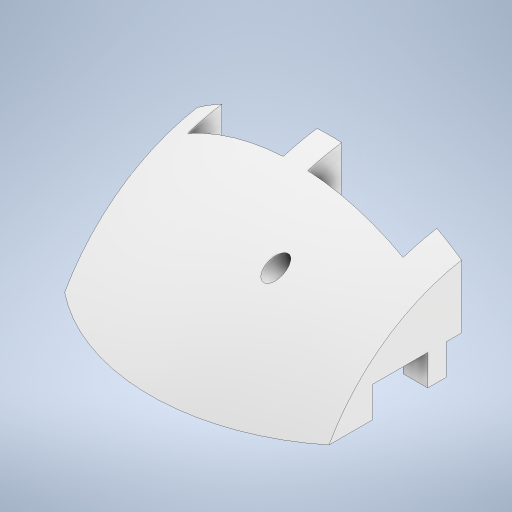
# Autodesk Inventor part: back back gabagaba
Saved by Autodesk Inventor 2023 (Build 270158000, 158)
## iProperties
Created: 2022-10-08
Part Number: back back gabagaba
Material: ABS プラスチック
Document SubType Name: Modeling
Designer: ellie
Density: 1.06 g/cm^3
Appearance: 積雪
Author: ellie
Autodesk Inventor part; units mm, degrees
sketch "スケッチ1" plane through (0, 0, 0) normal (0, 1, 0) x (-1, 0, 0)
  circle A0 centre (0, 0) radius 37.5
  line L0 (0, 0) -> (0, -37.5)
  line L1 (0, 0) -> (0, 37.5)
  dimension "d0" = 75
  constraints: 4 end point, 2 point on circle, 2 vertical, 1 centre point, 1 coincident
  measures "d0" diameter of A0
revolve "回転1" add sketch "スケッチ1" angle 180 about axis through (0, 0, 0) along (0, 0, 1) picked at (-2.7815, -24.6866) contours L1 L0 A0
sketch "スケッチ5" plane through (0, 0, 0) normal (0, -1, 0) x (1, 0, 0)
  line L0 (-21, -21) -> (21, -21)
  line L1 (21, -21) -> (21, -9)
  line L2 (21, -9) -> (-21, -9)
  line L3 (-21, -9) -> (-21, -21)
  line L4 (-21, -11) -> (-21, -9)
  line L5 (0, 25.75) -> (-17, 25.75)
  line L6 (-17, 25.75) -> (-17, 24.25)
  line L7 (-17, 24.25) -> (0, 24.25)
  line L8 (0, 24.25) -> (0, 25.75)
  line L9 (0, 22.75) -> (-20.5, 22.75)
  line L10 (-20.5, 22.75) -> (-20.5, 21.25)
  line L11 (-20.5, 21.25) -> (0, 21.25)
  line L12 (0, 21.25) -> (0, 22.75)
  line L13 (0, 15.75) -> (-21.5, 15.75)
  line L14 (-21.5, 15.75) -> (-21.5, 13.25)
  line L15 (-21.5, 13.25) -> (0, 13.25)
  line L16 (0, 13.25) -> (0, 15.75)
  line L17 (0, 7.75) -> (-22, 7.75)
  line L18 (-22, 7.75) -> (-22, 5.25)
  line L19 (-22, 5.25) -> (0, 5.25)
  line L20 (0, 5.25) -> (0, 7.75)
  circle A0 centre (0, 0) radius 37.5 projected
  circle A1 centre (0, 0) radius 37.5 projected
  line L21 (0, 37.5) -> (0, -37.5)
  line L22 (37.5, 0) -> (-37.5, 0)
  line L23 (-33.5, 5.25) -> (-24, 5.25)
  line L24 (-24, 5.25) -> (-24, -5.25)
  line L25 (-24, -5.25) -> (-33.5, -5.25)
  line L26 (-33.5, -5.25) -> (-33.5, 5.25)
  line L27 (-24, -8.0262) -> (-24, 5.25)
  line L28 (-29, 23.775) -> (-29, -23.775)
  line L29 (-14, 25.75) -> (0, 25.75)
  line L30 (0, 25.75) -> (0, 37.5)
  line L31 (-14, 37.5) -> (-14, 25.75)
  line L32 (-14, 24.25) -> (0, 24.25)
  line L33 (0, 24.25) -> (0, 22.75)
  line L34 (0, 22.75) -> (-14, 22.75)
  line L35 (-14, 22.75) -> (-14, 24.25)
  line L36 (-19, 15.75) -> (0, 15.75)
  line L37 (0, 15.75) -> (0, 21.25)
  line L38 (0, 21.25) -> (-19, 21.25)
  line L39 (-19, 21.25) -> (-19, 15.75)
  line L40 (-19, 13.25) -> (0, 13.25)
  line L41 (0, 13.25) -> (0, 7.75)
  line L42 (0, 7.75) -> (-19, 7.75)
  line L43 (-19, 7.75) -> (-19, 13.25)
  line L44 (-24, 0) -> (-40.9365, 0)
  line L45 (-24, 0) -> (-9.0837, 0)
  line L46 (-8.5, 5.25) -> (-24, 5.25)
  line L47 (-24, 5.25) -> (-24, -5.25)
  line L48 (-24, -5.25) -> (-8.5, -5.25)
  line L49 (-8.5, 5.25) -> (-24, -5.25) construction
  line L50 (-24, 5.25) -> (-8.5, -5.25) construction
  line L51 (-24, 7.25) -> (-34.5, 7.25)
  line L52 (-34.5, 7.25) -> (-34.5, -7.25)
  line L53 (-34.5, -7.25) -> (-24, -7.25)
  line L54 (-24, 7.25) -> (-34.5, -7.25) construction
  line L55 (-34.5, 7.25) -> (-24, -7.25) construction
  line L56 (-8.5, 5.25) -> (-1, 5.25)
  line L57 (-1, 5.25) -> (-1, -5.25)
  line L58 (-1, -5.25) -> (-8.5, -5.25)
  line L59 (-8.5, 5.25) -> (-1, -5.25) construction
  line L60 (-1, 5.25) -> (-8.5, -5.25) construction
  line L61 (-24, 5.25) -> (-29, 5.25)
  line L62 (-24, -5.25) -> (-29, -5.25)
  line L63 (-24, 7.25) -> (-29, 7.25)
  line L64 (-24, -7.25) -> (-29, -7.25)
  line L65 (27.0231, -26) -> (-27.0231, -26)
  line L66 (-8.5, 5.25) -> (-7.3, 5.25)
  line L67 (-7.3, -5.25) -> (-8.5, -5.25)
  line L68 (-4, 7.75) -> (-1, 7.75)
  line L69 (0, 22.75) -> (-4, 22.75)
  line L70 (-4, 21.25) -> (0, 21.25)
  line L71 (0, 21.25) -> (0, 22.75)
  line L72 (-7, 7.75) -> (-2, 7.75)
  line L73 (-1, 5.25) -> (-6.5, 5.25)
  line L74 (-24, 5.25) -> (-24, 7.25)
  point P0 (0, -21)
  point P1 (0, -9)
  point P2 (0, 25)
  point P3 (0, 22)
  point P4 (0, 14.5)
  point P5 (0, 6.5)
  point P6 (-21, -15)
  point P7 (-27, -0.5262)
  point P8 (-14, 23.5)
  point P9 (-14, 34.7886)
  point P10 (0, 25.75)
  point P11 (0, 24.25)
  point P12 (0, 13.25)
  point P13 (0, 15.75)
  point P14 (-29, 0)
  point P15 (-33.5, 0)
  point P16 (-24, 0)
  point P17 (-16.25, 0)
  point P18 (-29.25, 0)
  point P19 (-4.75, 0)
  point P20 (-27, 0.5)
  point P21 (-28, 0.4738)
  point P22 (-28, -11.5262)
  point P23 (-27, -11.5)
  point P24 (-24, 5.25)
  point P25 (-24, 5.25)
  point P26 (-1, 0)
  point P27 (0, 21.25)
  point P28 (0, 22.75)
  point P29 (-29, -7.25)
  point P30 (-29, 7.25)
  point P31 (-7.9, -5.25)
  point P32 (-7.9, 5.25)
  dimension "d12" = 42
  dimension "d13" = 12
  dimension "d23" = 17
  dimension "d24" = 1.5
  dimension "d27" = 20.5
  dimension "d28" = 1.5
  dimension "d30" = 21.5
  dimension "d31" = 2.5
  dimension "d33" = 2.5
  dimension "d88" = 0
  dimension "d89" = 0
  dimension "d90" = 16.5
  dimension "d92" = 21
  dimension "d97" = 9.5
  dimension "d98" = 10.5
  dimension "d113" = 29
  dimension "d122" = 14
  dimension "d124" = 1.5
  dimension "d125" = 14
  dimension "d126" = 5.5
  dimension "d127" = 5.5
  dimension "d128" = 19
  dimension "d129" = 19
  dimension "d161" = 14.5
  dimension "d162" = 10.5
  dimension "d164" = 10.5
  dimension "d170" = 26
  dimension "d326" = 23
  dimension "d327" = 10.5
  dimension "d329" = 15.5
  dimension "d330" = 34.5
  dimension "d359" = 22
  constraints: 148 end point, 26 parallel, 20 horizontal, 17 midpoint, 17 perpendicular, 16 point on line, 9 collinear, 2 vertical, 20 other
  measures "d12" distance of L2.end L1.end
  measures "d13" distance of L1.end L0.end
  measures "d23" distance of L7.end L6.end
  measures "d24" distance of L6.end L5.end
  measures "d27" distance of L11.end L10.end
  measures "d28" distance of L10.end L9.end
  measures "d30" distance of L15.end L14.end
  measures "d31" distance of L14.end L13.end
  measures "d33" distance of L18.end L17.end
  measures "d89" distance from line of point (0, 0) L22
  measures "d90" distance from line of L0 point (0, -37.5)
  measures "d92" distance of the line from the sketch origin of L3
  measures "d97" distance of L24.end L25.end
  measures "d98" distance of L23.end L24.end
  measures "d113" distance of the line from the sketch origin of L28
  measures "d122" distance of the line from the sketch origin of L31
  measures "d124" distance of L32.end L33.end
  measures "d126" distance of L37.end L36.end
  measures "d127" distance of L40.end L41.end
  measures "d128" distance of the line from the sketch origin of L43
  measures "d129" distance of the line from the sketch origin of L39
  measures "d161" distance between parallel lines of L53 L51
  measures "d162" distance between parallel lines of L47 L52
  measures "d164" distance between parallel lines of L58 L56
  measures "d170" distance between parallel lines of L65 L22
  measures "d326" distance between parallel lines of L47 L57
  measures "d327" distance between parallel lines of L48 L46
  measures "d329" distance of L47.end L48.end
  measures "d330" distance of the line from the sketch origin of L52
  measures "d359" distance of the line from the sketch origin of L18
extrude "GNSボード" cut sketch "スケッチ5" against normal blind 16 contours L8 L7 L6 L5
extrude "GNSボード止めるよう" cut sketch "スケッチ5" against normal blind 15 contours L21 L5 L31 A0 | L21 L9 L35 L7
extrude "アルミ板１" cut sketch "スケッチ5" against normal blind 20 contours L11 L10 L9 L12
extrude "メイン基板" cut sketch "スケッチ5" against normal blind 20 contours L15 L14 L13 L16
extrude "メイン止めるよう" cut sketch "スケッチ5" against normal blind 15 contours L17 L43 L15 L21 | L13 L39 L11 L21
extrude "アルミ板２" cut sketch "スケッチ5" against normal blind 20 contours L19 L18 L17 L20
extrude "電池ボックス入れ" cut sketch "スケッチ5" against normal blind 13 contours L3 L2 L21 L0 | L21 L2 L1 L0
extrude "side ut" cut sketch "スケッチ5" against normal blind 100 contours A0 L22 L52 L53 L28 | A0 L28 L51 L52 L22 | L53 L52 L22 L26 L25 L28 | L52 L51 L28 L23 L26 L22 | L25 L26 L22 L28 | L22 L26 L23 L28
extrude "motor case" add sketch "スケッチ5" against normal blind 7 contours L53 L52 L22 L26 L25 L28 | L24 L25 L28 L22 | L22 L28 L23 L24 | L52 L51 L28 L23 L26 L22 | L25 L26 L22 L28 | L22 L26 L23 L28
extrude "bottom cut" cut sketch "スケッチ5" against normal blind 90 contours L65 A0 L21 | L21 A0 L65
extrude "motor" cut sketch "スケッチ5" against normal blind 6 contours L57 L58 L48 L24 L22 | L22 L24 L46 L19 L57 | L24 L25 L28 L22 | L22 L28 L23 L24 | L25 L26 L22 L28 | L22 L26 L23 L28
sketch "スケッチ27" plane through (-34.5, 0, -7.25) normal (-1, 0, 0) x (0, 0, 1)
  line L0 (14.5, 0) -> (0, 0) projected
  circle A0 centre (7.25, 0) radius 3
  point P0 (7.25, 0)
  dimension "d198" = 6
  constraints: 1 centre point, 1 midpoint
  measures "d198" diameter of A0
extrude "moter shaft" cut sketch "スケッチ27" against normal blind 27
mirror "ミラー13" about plane through (0, 0, 0) normal (1, 0, 0) of "メイン止めるよう", "メイン基板", "アルミ板１", "GNSボード止めるよう", "GNSボード", "アルミ板２", "motor", "motor case", "moter shaft", "電池ボックス入れ", "side ut"
ref_plane "作業平面5" through (-17, 17.5, 24.25) normal (0, -1, 0) x (1, 0, 0)
ref_plane "作業平面6" through (21, 13, -9) normal (0, 0, -1) x (1, 0, 0)
ref_plane "作業平面7" through (29, 35, 7.25) normal (0, -1, 0) x (1, 0, 0)
sketch "スケッチ41" plane through (-17, 0, 24.25) normal (0, -1, 0) x (1, 0, 0)
  line L0 (-17.5, -21.25) -> (-16.5, -21.25) projected
  line L1 (-16.5, -21.25) -> (-16.5, -19) projected
  line L2 (-16.5, -19) -> (-5, -19) projected
  line L3 (-5, -19) -> (-5, -16.5) projected
  line L4 (-5, -16.5) -> (-2, -16.5) projected
  line L5 (-2, -16.5) -> (-2, -11) projected
  line L6 (-2, -11) -> (-4.5, -11) projected
  line L7 (-4.5, -11) -> (-4.5, -8.5) projected
  line L8 (-4.5, -8.5) -> (-2, -8.5) projected
  line L9 (-2, -8.5) -> (-2, -3) projected
  line L10 (-2, -3) -> (-3.5, -3) projected
  line L11 (-3.5, -3) -> (-3.5, -1.5) projected
  line L12 (-3.5, -1.5) -> (3, -1.5) projected
  line L13 (3, -1.5) -> (3, 0) projected
  line L14 (3, 0) -> (0, 0) projected
  line L15 (0, 0) -> (0, 1.5) projected
  line L16 (0, 1.5) -> (3, 1.5) projected
  line L17 (3, 1.5) -> (3, 10.5386) projected
  arc A0 (3, 10.5386) -> (-12, -0.475) centre (17, -24.25) ccw projected
  line L18 (-12, -0.475) -> (-12, -17) projected
  line L19 (-12, -17) -> (-17.5, -17) projected
  line L20 (-17.5, -17) -> (-17.5, -21.25) projected
  line L21 (-2, -16.5) -> (-2, -11) projected
  line L22 (-4.5, -8.5) -> (-4.5, -11) projected
  line L23 (0, 1.5) -> (0, 0) projected
  circle A1 centre (-4.5, 2.5) radius 2.25
  dimension "d252" = 4.5
  dimension "d253" = 4.5
  dimension "d254" = 4
  constraints: 1 centre point
  measures "d252" diameter of A1
  measures "d253" distance from line of A1.centre L15
  measures "d254" distance from line of A1.centre L12
extrude "top lock 10mm" cut sketch "スケッチ41" against normal blind 3 contours A1
mirror "ミラー15" about plane through (0, 0, 0) normal (1, 0, 0) of "top lock 10mm"
sketch "スケッチ42" plane through (-34.5, 0, -7.25) normal (0, -1, 0) x (1, 0, 0)
  circle A0 centre (9.5, -14) radius 2.25
  line L0 (13.5, -13.75) -> (13.5, -1.75) projected
  line L1 (33.5, 2) -> (1, 2) projected
  point P0 (34.5, 7.25)
  point P1 (10, 2)
  point P2 (7.8183, 2)
  point P3 (12.1817, 2)
  dimension "d257" = 4
  dimension "d258" = 4.5
  dimension "d259" = 16
  constraints: 1 centre point
  measures "d257" distance from line of A0.centre L0
  measures "d258" diameter of A0
  measures "d259" distance from line of A0.centre L1
extrude "bottom lock" cut sketch "スケッチ42" against normal blind 3
mirror "ミラー16" about plane through (0, 0, 0) normal (1, 0, 0) of "bottom lock"
ref_plane "作業平面8" through (-17, 15, 24.25) normal (0, -1, 0) x (1, 0, 0)
sketch "スケッチ45" plane through (-17, 15, 24.25) normal (0, -1, 0) x (1, 0, 0)
  circle A0 centre (-4.5, 2.5) radius 2.25 projected
  line L0 (-17.5, -21.25) -> (-16.5, -21.25) projected
  line L1 (-16.5, -21.25) -> (-16.5, -19) projected
  line L2 (-16.5, -19) -> (-5, -19) projected
  line L3 (-5, -19) -> (-5, -16.5) projected
  line L4 (-5, -16.5) -> (-2, -16.5) projected
  line L5 (-2, -16.5) -> (-2, -11) projected
  line L6 (-2, -11) -> (-4.5, -11) projected
  line L7 (-4.5, -11) -> (-4.5, -8.5) projected
  line L8 (-4.5, -8.5) -> (-2, -8.5) projected
  line L9 (-2, -8.5) -> (-2, -3) projected
  line L10 (-2, -3) -> (-3.5, -3) projected
  line L11 (-3.5, -3) -> (-3.5, -1.5) projected
  line L12 (-3.5, -1.5) -> (3, -1.5) projected
  line L13 (3, -1.5) -> (3, 0) projected
  line L14 (3, 0) -> (0, 0) projected
  line L15 (0, 0) -> (0, 1.5) projected
  line L16 (0, 1.5) -> (3, 1.5) projected
  line L17 (3, 1.5) -> (3, 10.5386) projected
  arc A1 (3, 10.5386) -> (-12, -0.475) centre (17, -24.25) ccw projected
  line L18 (-12, -0.475) -> (-12, -17) projected
  line L19 (-12, -17) -> (-17.5, -17) projected
  line L20 (-17.5, -17) -> (-17.5, -21.25) projected
  arc A2 (31, 7.1387) -> (3, 7.1387) centre (17, -24.25) ccw projected
  line L21 (3, 1.5) -> (3, 7.1387) projected
  line L22 (31, 1.5) -> (3, 1.5) projected
  line L23 (31, 1.5) -> (31, 7.1387) projected
  circle A3 centre (38.5, 2.5) radius 2.25 projected
  line L24 (50.5, -21.25) -> (51.5, -21.25) projected
  line L25 (51.5, -17) -> (51.5, -21.25) projected
  line L26 (46, -17) -> (51.5, -17) projected
  line L27 (46, -17) -> (46, -0.475) projected
  arc A4 (46, -0.475) -> (31, 10.5386) centre (17, -24.25) ccw projected
  line L28 (31, 10.5386) -> (31, 1.5) projected
  line L29 (31, 1.5) -> (34, 1.5) projected
  line L30 (34, 1.5) -> (34, 0) projected
  line L31 (34, 0) -> (31, 0) projected
  line L32 (31, 0) -> (31, -1.5) projected
  line L33 (31, -1.5) -> (37.5, -1.5) projected
  line L34 (37.5, -1.5) -> (37.5, -3) projected
  line L35 (37.5, -3) -> (36, -3) projected
  line L36 (36, -3) -> (36, -8.5) projected
  line L37 (36, -8.5) -> (38.5, -8.5) projected
  line L38 (38.5, -8.5) -> (38.5, -11) projected
  line L39 (38.5, -11) -> (36, -11) projected
  line L40 (36, -11) -> (36, -16.5) projected
  line L41 (36, -16.5) -> (39, -16.5) projected
  line L42 (39, -16.5) -> (39, -19) projected
  line L43 (39, -19) -> (50.5, -19) projected
  line L44 (50.5, -19) -> (50.5, -21.25) projected
  circle A5 centre (38.5, 2.5) radius 2.25 projected
  arc A6 (-17.5, -21.25) -> (-17.5, -21.25) centre (-4.5, 2.5) ccw projected
  line L45 (34, 0) -> (0, 0) projected
  line L46 (34, 0) -> (34, 1.5) projected
  line L47 (34, 1.5) -> (0, 1.5) projected
  line L48 (0, 0) -> (0, 1.5) projected
  line L49 (31, -1.5) -> (3, -1.5) projected
  line L50 (31, -1.5) -> (31, 0) projected
  line L51 (3, 0) -> (31, 0) projected
  line L52 (3, -1.5) -> (3, 0) projected
  line L53 (-2, -3) -> (36, -3) projected
  arc A7 (50.5, -21.25) -> (50.5, -21.25) centre (38.5, 2.5) ccw projected
  line L54 (36, -8.5) -> (-2, -8.5) projected
  line L55 (36, -8.5) -> (36, -3) projected
  line L56 (-2, -3) -> (36, -3) projected
  line L57 (-2, -8.5) -> (-2, -3) projected
  line L58 (-2, -11) -> (36, -11) projected
  line L59 (36, -16.5) -> (-2, -16.5) projected
  line L60 (36, -16.5) -> (36, -11) projected
  line L61 (-2, -11) -> (36, -11) projected
  line L62 (-2, -16.5) -> (-2, -11) projected
  line L63 (39, -19) -> (-5, -19) projected
  line L64 (39, -19) -> (39, -16.5) projected
  line L65 (39, -16.5) -> (-5, -16.5) projected
  line L66 (-5, -19) -> (-5, -16.5) projected
  line L67 (-5, -19) -> (16, -19) projected
  line L68 (-16.5, -19) -> (-5, -19) projected
  line L69 (-16.5, -29.5) -> (-16.5, -19) projected
  line L70 (16, -29.5) -> (-16.5, -29.5) projected
  circle A8 centre (42, -45.5) radius 2.25 projected
  circle A9 centre (-8, -45.5) radius 2.25 projected
  line L71 (18, -29.5) -> (18, -19) projected
  line L72 (18, -19) -> (16, -19) projected
  line L73 (16, -19) -> (16, -29.5) projected
  line L74 (-5, -19) -> (-5, -16.5) projected
  line L75 (-16.5, -29.5) -> (-16.5, -27.25) projected
  line L76 (-16.5, -27.25) -> (-17.5, -27.25) projected
  line L77 (-17.5, -27.25) -> (-17.5, -31.5) projected
  line L78 (-17.5, -31.5) -> (-12, -31.5) projected
  line L79 (-12, -31.5) -> (-12, -48.025) projected
  arc A10 (-12, -48.025) -> (-10.0231, -50.25) centre (17, -24.25) ccw projected
  line L80 (-10.0231, -50.25) -> (44.0231, -50.25) projected
  arc A11 (44.0231, -50.25) -> (46, -48.025) centre (17, -24.25) ccw projected
  line L81 (46, -48.025) -> (46, -31.5) projected
  line L82 (51.5, -31.5) -> (46, -31.5) projected
  line L83 (51.5, -27.25) -> (51.5, -31.5) projected
  line L84 (51.5, -27.25) -> (50.5, -27.25) projected
  line L85 (50.5, -27.25) -> (50.5, -29.5) projected
  line L86 (39, -16.5) -> (39, -19) projected
  line L87 (-4, -33.25) -> (38, -33.25) projected
  line L88 (38, -33.25) -> (38, -45.25) projected
  line L89 (38, -45.25) -> (-4, -45.25) projected
  line L90 (-4, -45.25) -> (-4, -33.25) projected
  line L91 (-5, -13.5) -> (39, -13.5)
  line L92 (39, -13.5) -> (39, 10.1193)
  line L93 (39, 10.1193) -> (-5, 10.1193)
  line L94 (-5, 10.1193) -> (-5, -13.5)
  line L95 (16, -19) -> (16, -29.5) projected
  line L96 (-17.5, -21.25) -> (-16.5, -21.25) projected
  line L97 (-16.5, -21.25) -> (-16.5, -19) projected
  line L98 (-16.5, -19) -> (-5, -19) projected
  line L99 (-5, -16.5) -> (-2, -16.5) projected
  line L100 (-2, -16.5) -> (-2, -11) projected
  line L101 (-2, -11) -> (-4.5, -11) projected
  line L102 (-4.5, -11) -> (-4.5, -8.5) projected
  line L103 (-4.5, -8.5) -> (-2, -8.5) projected
  line L104 (-2, -8.5) -> (-2, -3) projected
  line L105 (-2, -3) -> (-3.5, -3) projected
  line L106 (-3.5, -3) -> (-3.5, -1.5) projected
  line L107 (-3.5, -1.5) -> (3, -1.5) projected
  line L108 (3, -1.5) -> (3, 0) projected
  line L109 (3, 0) -> (0, 0) projected
  line L110 (0, 0) -> (0, 1.5) projected
  line L111 (0, 1.5) -> (3, 1.5) projected
  line L112 (3, 1.5) -> (3, 10.5386) projected
  line L113 (-12, -0.475) -> (-12, -17) projected
  line L114 (-12, -17) -> (-17.5, -17) projected
  line L115 (-17.5, -17) -> (-17.5, -21.25) projected
  line L116 (16, -29.5) -> (-16.5, -29.5) projected
  line L117 (50.5, -29.5) -> (18, -29.5) projected
  line L118 (50.5, -21.25) -> (51.5, -21.25) projected
  line L119 (51.5, -17) -> (51.5, -21.25) projected
  line L120 (46, -17) -> (51.5, -17) projected
  line L121 (46, -17) -> (46, -0.475) projected
  line L122 (31, 10.5386) -> (31, 1.5) projected
  line L123 (31, 1.5) -> (34, 1.5) projected
  line L124 (34, 1.5) -> (34, 0) projected
  line L125 (34, 0) -> (31, 0) projected
  line L126 (31, 0) -> (31, -1.5) projected
  line L127 (31, -1.5) -> (37.5, -1.5) projected
  line L128 (37.5, -1.5) -> (37.5, -3) projected
  line L129 (37.5, -3) -> (36, -3) projected
  line L130 (36, -3) -> (36, -8.5) projected
  line L131 (36, -8.5) -> (38.5, -8.5) projected
  line L132 (38.5, -8.5) -> (38.5, -11) projected
  line L133 (38.5, -11) -> (36, -11) projected
  line L134 (36, -11) -> (36, -16.5) projected
  line L135 (36, -16.5) -> (39, -16.5) projected
  line L136 (39, -19) -> (50.5, -19) projected
  line L137 (50.5, -19) -> (50.5, -21.25) projected
  arc A12 (3, 10.5386) -> (-12, -0.475) centre (17, -24.25) ccw projected
  arc A13 (46, -0.475) -> (31, 10.5386) centre (17, -24.25) ccw projected
  arc A14 (44.0231, -50.25) -> (46, -48.025) centre (17, -24.25) ccw projected
  arc A15 (-12, -48.025) -> (-10.0231, -50.25) centre (17, -24.25) ccw projected
  circle A16 centre (-4.5, 2.5) radius 2.25 projected
  circle A17 centre (38.5, 2.5) radius 2.25 projected
  line L138 (51.5, -27.25) -> (50.5, -27.25) projected
  line L139 (50.5, -29.5) -> (18, -29.5) projected
  line L140 (18, -29.5) -> (18, -19) projected
  line L141 (18, -19) -> (16, -19) projected
  line L142 (16, -19) -> (16, -29.5) projected
  line L143 (16, -29.5) -> (-16.5, -29.5) projected
  line L144 (-17.5, -21.25) -> (-16.5, -21.25) projected
  line L145 (-16.5, -27.25) -> (-17.5, -27.25) projected
  line L146 (-16.5, -29.5) -> (-16.5, -27.25) projected
  line L147 (-17.5, -27.25) -> (-17.5, -31.5) projected
  line L148 (-17.5, -31.5) -> (-12, -31.5) projected
  line L149 (-12, -31.5) -> (-12, -48.025) projected
  arc A18 (-12, -48.025) -> (-10.0231, -50.25) centre (17, -24.25) ccw projected
  line L150 (-10.0231, -50.25) -> (44.0231, -50.25) projected
  line L151 (46, -48.025) -> (46, -31.5) projected
  line L152 (51.5, -31.5) -> (46, -31.5) projected
  line L153 (51.5, -27.25) -> (51.5, -31.5) projected
  line L154 (50.5, -27.25) -> (50.5, -29.5) projected
  line L155 (51.5, -27.25) -> (50.5, -27.25) projected
  line L156 (50.5, -21.25) -> (51.5, -21.25) projected
  line L157 (50.5, -29.5) -> (18, -29.5) projected
  line L158 (18, -29.5) -> (18, -19) projected
  line L159 (18, -19) -> (16, -19) projected
  line L160 (16, -19) -> (16, -29.5) projected
  line L161 (16, -29.5) -> (-16.5, -29.5) projected
  line L162 (-16.5, -27.25) -> (-17.5, -27.25) projected
  line L163 (-16.5, -29.5) -> (-16.5, -27.25) projected
  line L164 (-17.5, -27.25) -> (-17.5, -31.5) projected
  line L165 (-17.5, -31.5) -> (-12, -31.5) projected
  line L166 (-12, -31.5) -> (-12, -48.025) projected
  line L167 (-10.0231, -50.25) -> (44.0231, -50.25) projected
  arc A19 (44.0231, -50.25) -> (46, -48.025) centre (17, -24.25) ccw projected
  line L168 (46, -48.025) -> (46, -31.5) projected
  line L169 (51.5, -31.5) -> (46, -31.5) projected
  line L170 (51.5, -27.25) -> (51.5, -31.5) projected
  line L171 (50.5, -27.25) -> (50.5, -29.5) projected
  line L172 (-16.5, -21.25) -> (-16.5, -19) projected
  line L173 (-16.5, -19) -> (-5, -19) projected
  line L174 (-5, -19) -> (-5, -16.5) projected
  line L175 (-5, -16.5) -> (-2, -16.5) projected
  line L176 (-2, -16.5) -> (-2, -11) projected
  line L177 (-2, -11) -> (-4.5, -11) projected
  line L178 (-4.5, -11) -> (-4.5, -8.5) projected
  line L179 (-4.5, -8.5) -> (-2, -8.5) projected
  line L180 (-2, -8.5) -> (-2, -3) projected
  line L181 (-2, -3) -> (-3.5, -3) projected
  line L182 (-3.5, -3) -> (-3.5, -1.5) projected
  line L183 (-3.5, -1.5) -> (3, -1.5) projected
  line L184 (3, -1.5) -> (3, 0) projected
  line L185 (3, 0) -> (0, 0) projected
  line L186 (0, 0) -> (0, 1.5) projected
  line L187 (0, 1.5) -> (3, 1.5) projected
  line L188 (3, 1.5) -> (3, 10.5386) projected
  arc A20 (3, 10.5386) -> (-12, -0.475) centre (17, -24.25) ccw projected
  line L189 (-12, -0.475) -> (-12, -17) projected
  line L190 (-12, -17) -> (-17.5, -17) projected
  line L191 (-17.5, -17) -> (-17.5, -21.25) projected
  line L192 (51.5, -17) -> (51.5, -21.25) projected
  line L193 (46, -17) -> (51.5, -17) projected
  line L194 (46, -17) -> (46, -0.475) projected
  arc A21 (46, -0.475) -> (31, 10.5386) centre (17, -24.25) ccw projected
  line L195 (31, 10.5386) -> (31, 1.5) projected
  line L196 (31, 1.5) -> (34, 1.5) projected
  line L197 (34, 1.5) -> (34, 0) projected
  line L198 (34, 0) -> (31, 0) projected
  line L199 (31, 0) -> (31, -1.5) projected
  line L200 (31, -1.5) -> (37.5, -1.5) projected
  line L201 (37.5, -1.5) -> (37.5, -3) projected
  line L202 (37.5, -3) -> (36, -3) projected
  line L203 (36, -3) -> (36, -8.5) projected
  line L204 (36, -8.5) -> (38.5, -8.5) projected
  line L205 (38.5, -8.5) -> (38.5, -11) projected
  line L206 (38.5, -11) -> (36, -11) projected
  line L207 (36, -11) -> (36, -16.5) projected
  line L208 (36, -16.5) -> (39, -16.5) projected
  line L209 (39, -16.5) -> (39, -19) projected
  line L210 (39, -19) -> (50.5, -19) projected
  line L211 (50.5, -19) -> (50.5, -21.25) projected
  line L212 (-2, -3) -> (36, -3) projected
  line L213 (-2, -8.5) -> (-2, -3) projected
  line L214 (36, -8.5) -> (-2, -8.5) projected
  line L215 (36, -8.5) -> (36, -3) projected
  line L216 (-2, -11) -> (36, -11) projected
  line L217 (-2, -16.5) -> (-2, -11) projected
  line L218 (36, -16.5) -> (-2, -16.5) projected
  line L219 (36, -16.5) -> (36, -11) projected
  dimension "d269" = 3
  constraints: 8 end point, 2 collinear, 2 parallel, 1 horizontal, 1 perpendicular, 1 tangent, 2 other
  measures "d269" distance between parallel lines of L91 L65
extrude "back cut" cut sketch "スケッチ45" along normal blind 25 contours A0 L94 | A0 L94 A1 L93 L17 L16 L15 L14 L13 L12 L11 L10 L9 L8 L7 L6 L5 L91 | L94 L93 A1 | L5 L58 A7 L91 | L93 A7 A2 L17 | L6 L7 L8 L54 A7 L58 | A7 L58 A6 L91 | A2 A7 L22 L17 | L93 A2 A7 | A7 L54 A6 L58 | A6 L58 L40 L91 | L22 A7 L45 L14 L15 L16 | A2 A6 L22 A7 | L93 A6 A2 | L54 L9 L53 A7 | A7 L53 A6 L54 | A6 L54 L37 L38 L39 L58 | L40 L39 L38 L37 L36 L35 L34 L33 L32 L31 L30 L29 L23 L28 L93 A4 L92 A3 L91 | L22 A6 L45 A7 | L93 L28 A2 A6 | A2 L23 L22 A6 | A7 L49 A6 L53 | L53 L10 L11 L12 L49 A7 | A6 L53 L36 L54 | L22 L29 L30 L31 L45 A6 | A7 L49 L13 L45 | L45 A6 L49 A7 | A6 L49 L33 L34 L35 L53 | A3 L92 | L45 L32 L49 A6 | L93 L92 A4 picked at (-4.1021, 2.6669) picked at (38.0887, 2.5895)
ref_plane "作業平面11" through (0, 13, 0) normal (0, -1, 0) x (1, 0, 0)
sketch "スケッチ71" plane through (-22, 0, 7.75) normal (0, -1, 0) x (1, 0, 0)
  line L0 (0, -2.5) -> (0, 0) projected
  line L1 (0, -2.5) -> (44, -2.5)
  line L2 (44, -2.5) -> (44, 26.6193)
  line L3 (44, 26.6193) -> (0, 26.6193)
  line L4 (0, 26.6193) -> (0, -2.5)
  line L5 (44, 16.8063) -> (44, 3) projected
  arc A0 (44, 18.6555) -> (0, 18.6555) centre (22, -7.75) ccw projected
  line L6 (0, 21.1937) -> (0, 22.6186) projected
  arc A1 (0, 22.6186) -> (-7, 16.025) centre (22, -7.75) ccw projected
  line L7 (-7, 16.025) -> (-7, -0.5) projected
  line L8 (-7, -0.5) -> (-12.5, -0.5) projected
  line L9 (-12.5, -0.5) -> (-12.5, -4.75) projected
  line L10 (-12.5, -4.75) -> (-11.5, -4.75) projected
  line L11 (-11.5, -4.75) -> (-11.5, -2.5) projected
  line L12 (-11.5, -2.5) -> (0, -2.5) projected
  line L13 (0, -2.5) -> (0, 0) projected
  line L14 (0, 0) -> (3, 0) projected
  line L15 (3, 0) -> (3, 3) projected
  line L16 (3, 3) -> (0, 3) projected
  line L17 (0, 3) -> (0, 16.8063) projected
  arc A2 (0, 21.1937) -> (0, 16.8063) centre (0.5, 19) ccw projected
  circle A3 centre (47, -29) radius 2.25 projected
  circle A4 centre (-3, -29) radius 2.25 projected
  line L18 (1, -16.75) -> (43, -16.75) projected
  line L19 (43, -16.75) -> (43, -28.75) projected
  line L20 (43, -28.75) -> (1, -28.75) projected
  line L21 (1, -28.75) -> (1, -16.75) projected
  line L22 (56.5, -10.75) -> (55.5, -10.75) projected
  line L23 (55.5, -10.75) -> (55.5, -13) projected
  line L24 (55.5, -13) -> (23, -13) projected
  line L25 (23, -13) -> (23, -2.5) projected
  line L26 (23, -2.5) -> (21, -2.5) projected
  line L27 (21, -2.5) -> (21, -13) projected
  line L28 (21, -13) -> (-11.5, -13) projected
  line L29 (-11.5, -13) -> (-11.5, -10.75) projected
  line L30 (-11.5, -10.75) -> (-12.5, -10.75) projected
  line L31 (-12.5, -10.75) -> (-12.5, -15) projected
  line L32 (-12.5, -15) -> (-7, -15) projected
  line L33 (-7, -15) -> (-7, -31.525) projected
  arc A5 (-7, -31.525) -> (-5.0231, -33.75) centre (22, -7.75) ccw projected
  line L34 (-5.0231, -33.75) -> (49.0231, -33.75) projected
  arc A6 (49.0231, -33.75) -> (51, -31.525) centre (22, -7.75) ccw projected
  line L35 (51, -31.525) -> (51, -15) projected
  line L36 (56.5, -15) -> (51, -15) projected
  line L37 (56.5, -10.75) -> (56.5, -15) projected
  line L38 (44, 22.6186) -> (44, 21.1937) projected
  arc A7 (44, 16.8063) -> (44, 21.1937) centre (43.5, 19) ccw projected
  line L39 (44, 16.8063) -> (44, 3) projected
  line L40 (44, 3) -> (41, 3) projected
  line L41 (41, 3) -> (41, 0) projected
  line L42 (41, 0) -> (44, 0) projected
  line L43 (44, 0) -> (44, -2.5) projected
  line L44 (44, -2.5) -> (55.5, -2.5) projected
  line L45 (55.5, -2.5) -> (55.5, -4.75) projected
  line L46 (55.5, -4.75) -> (56.5, -4.75) projected
  line L47 (56.5, -0.5) -> (56.5, -4.75) projected
  line L48 (51, -0.5) -> (56.5, -0.5) projected
  line L49 (51, -0.5) -> (51, 16.025) projected
  arc A8 (51, 16.025) -> (44, 22.6186) centre (22, -7.75) ccw projected
  point P0 (21, -2.5)
  point P1 (44, -2.5)
  point P2 (0, -2.5)
  constraints: 8 end point, 2 parallel, 1 collinear, 1 horizontal, 1 perpendicular, 1 tangent
extrude "押し出し69" cut sketch "スケッチ71" against normal blind 50 contours L12 L11 L10 L9 L8 L7 A1 L4 A2 L0 | L1 L25 L24 L23 L22 L37 L36 L35 A6 L34 A5 L33 L32 L31 L30 L29 L28 L27 | A2 L4 | L2 A7 A8 L49 L48 L47 L46 L45 L44 | L2 A7 | A3 | A4 | L18 L19 L20 L21
sketch "スケッチ73" plane through (0, 15, 0) normal (0, -1, 0) x (1, 0, 0)
  point P0 (0, 0)
sketch "バック切り出しスケッチ" plane through (0, 15, 0) normal (0, -1, 0) x (1, 0, 0)
  line L0 (22, 5.25) -> (1, 5.25) projected
  line L1 (22, 5.25) -> (22, 7.75) projected
  line L2 (22, 7.75) -> (-22, 7.75) projected
  line L3 (-22, 5.25) -> (-22, 7.75) projected
  line L4 (-1, 5.25) -> (-22, 5.25) projected
  line L5 (1, 5.25) -> (-1, 5.25) projected
  line L6 (20.5, 21.25) -> (20.5, 22.75) projected
  line L7 (-20.5, 21.25) -> (20.5, 21.25) projected
  line L8 (-20.5, 22.75) -> (-20.5, 21.25) projected
  line L9 (20.5, 22.75) -> (-20.5, 22.75) projected
  arc A0 (22, 26.4055) -> (-22, 26.4055) centre (0, 0) ccw projected
  line L10 (-22, 26.4055) -> (-22, 10.75) projected
  line L11 (-22, 10.75) -> (-19, 10.75) projected
  line L12 (-19, 7.75) -> (-19, 10.75) projected
  line L13 (19, 7.75) -> (-19, 7.75) projected
  line L14 (19, 7.75) -> (19, 10.75) projected
  line L15 (19, 10.75) -> (22, 10.75) projected
  line L16 (22, 10.75) -> (22, 26.4055) projected
  line L17 (17, 25.75) -> (-17, 25.75) projected
  line L18 (17, 24.25) -> (17, 25.75) projected
  line L19 (-17, 24.25) -> (17, 24.25) projected
  line L20 (-17, 25.75) -> (-17, 24.25) projected
  line L21 (-22, 5.25) -> (22, 5.25)
  line L22 (22, 5.25) -> (22, 38.0096)
  line L23 (22, 38.0096) -> (-22, 38.0096)
  line L24 (-22, 38.0096) -> (-22, 5.25)
  line L25 (-43.9387, 44.3556) -> (43.0477, 44.3556)
  line L26 (43.0477, 44.3556) -> (43.0477, -31.2918)
  line L27 (43.0477, -31.2918) -> (-43.9387, -31.2918)
  line L28 (-43.9387, -31.2918) -> (-43.9387, 44.3556)
  point P0 (-22, 26.4055)
  point P1 (22, 26.4055)
  dimension "d373" = 86.9864
  dimension "d374" = 75.6474
  dimension "d375" = 6.346
  dimension "d376" = 21.0477
  dimension "d377" = 32.7596
  constraints: 16 end point, 4 parallel, 2 horizontal, 2 perpendicular, 1 collinear
  measures "d373" distance between parallel lines of L28 L26
  measures "d374" distance between parallel lines of L27 L25
  measures "d375" distance between parallel lines of L23 L25
  measures "d376" distance between parallel lines of L26 L22
  measures "d377" distance between parallel lines of L4 L23
extrude "バック切り取り押し出し１" cut sketch "バック切り出しスケッチ" along normal blind 50 contours L2 L14 L15 L22 | L2 L12 L11 L10 A0 L16 L15 L14 | L2 L24 L11 L12 | A0 L24 L23 L22 | L7 L8 L9 L6
extrude "バック切り取り押し出し２" cut sketch "バック切り出しスケッチ" along normal mid plane 50 contours L25 L26 L27 L28
sketch "スケッチ75" plane through (0, 0, 5.25) normal (0, 0, -1) x (-1, 0, 0)
  arc A0 (22, 29.9113) -> (-22, 29.9113) centre (0, 0) ccw projected
  line L0 (-22, 20) -> (-22, 29.9113) projected
  line L1 (-22, 20) -> (22, 20) projected
  line L2 (22, 20) -> (22, 29.9113) projected
  line L3 (-22, 15) -> (22, 15) projected
  line L4 (22, 15) -> (22, 20) projected
  line L5 (-22, 20) -> (22, 20) projected
  line L6 (-22, 15) -> (-22, 20) projected
  line L7 (22, 15) -> (17, 15)
  line L8 (17, 15) -> (17, 43.8577)
  line L9 (17, 43.8577) -> (22, 43.8577)
  line L10 (22, 43.8577) -> (22, 15)
  line L11 (2.5, 15) -> (-2.5, 15)
  line L12 (-2.5, 15) -> (-2.5, 43.8577)
  line L13 (-2.5, 43.8577) -> (2.5, 43.8577)
  line L14 (2.5, 43.8577) -> (2.5, 15)
  line L15 (17, 15) -> (-17, 15) projected
  line L16 (-17, 15) -> (-22, 15)
  line L17 (-22, 15) -> (-22, 42.8454)
  line L18 (-22, 42.8454) -> (-17, 42.8454)
  line L19 (-17, 42.8454) -> (-17, 15)
  line L20 (0, 15) -> (0, 37.1307)
  point P0 (-22, 28.9227)
  point P1 (-2.5, 37.0464)
  point P2 (-17, 33.0104)
  point P3 (2.5, 37.0464)
  point P4 (17, 15)
  point P5 (17, 33.0104)
  dimension "d380" = 0
  dimension "d381" = 5
  dimension "d382" = 5
  dimension "d383" = 2.5
  dimension "d384" = 5
  constraints: 26 end point, 6 parallel, 3 horizontal, 3 perpendicular, 3 point on line, 2 midpoint, 1 point on circle
  measures "d380" distance from line of point (-22, 28.923) L0
  measures "d381" distance between parallel lines of L17 L19
  measures "d382" distance between parallel lines of L14 L12
  measures "d383" distance between parallel lines of L14 L20
  measures "d384" distance between parallel lines of L2 L8
extrude "バック切り取り押し出し３" cut sketch "スケッチ75" against normal blind 5.5 contours L8 L1 L14 A0 | L8 L3 L14 L1 | L12 L1 L19 A0 | L12 L3 L19 L1
sketch "スケッチ78" plane through (0, 15, 0) normal (0, -1, 0) x (1, 0, 0)
  line L0 (17, 25.75) -> (-17, 25.75) projected
  line L1 (17, 24.25) -> (17, 25.75) projected
  line L2 (-17, 24.25) -> (17, 24.25) projected
  line L3 (-17, 25.75) -> (-17, 24.25) projected
  line L4 (-21.5, 13.25) -> (21.5, 13.25) projected
  line L5 (-21.5, 15.75) -> (-21.5, 13.25) projected
  line L6 (21.5, 15.75) -> (-21.5, 15.75) projected
  line L7 (21.5, 13.25) -> (21.5, 15.75) projected
  line L8 (20.5, 22.75) -> (-20.5, 22.75) projected
  line L9 (20.5, 21.25) -> (20.5, 22.75) projected
  line L10 (-20.5, 21.25) -> (20.5, 21.25) projected
  line L11 (-20.5, 22.75) -> (-20.5, 21.25) projected
  line L12 (2.5, 7.75) -> (2.5, 10.75) projected
  line L13 (2.5, 10.75) -> (17, 10.75) projected
  line L14 (17, 10.75) -> (17, 7.75) projected
  line L15 (22, 7.75) -> (17, 7.75) projected
  line L16 (22, 7.75) -> (22, 26.4055) projected
  arc A0 (22, 26.4055) -> (-22, 26.4055) centre (0, 0) ccw projected
  line L17 (-22, 26.4055) -> (-22, 7.75) projected
  line L18 (-17, 7.75) -> (-22, 7.75) projected
  line L19 (-17, 7.75) -> (-17, 10.75) projected
  line L20 (-17, 10.75) -> (-2.5, 10.75) projected
  line L21 (-2.5, 10.75) -> (-2.5, 7.75) projected
  line L22 (2.5, 7.75) -> (-2.5, 7.75) projected
  line L23 (-17, 10.75) -> (-22, 10.75)
  line L24 (-22, 10.75) -> (22, 10.75)
  line L25 (22, 10.75) -> (22, 19.75)
  line L26 (22, 19.75) -> (-22, 19.75)
  line L27 (-22, 19.75) -> (-22, 10.75)
  point P0 (-2.5, 10.75)
  dimension "d392" = 0
  dimension "d393" = 1.5
  constraints: 10 end point, 2 parallel, 2 perpendicular, 1 horizontal, 1 point on line
  measures "d392" distance between parallel lines of L16 L25
  measures "d393" distance between parallel lines of L26 L10
extrude "メイン基板ピッタリ用押しだし" cut sketch "スケッチ78" against normal up to surface (5 mm away) contours L24 L20 L23 L17 L26 L16 L13
sketch "がばがば用スケッチ" plane through (0, 15, 0) normal (0, -1, 0) x (1, 0, 0)
  line L0 (-22, 19.75) -> (22, 19.75) projected
  line L1 (22, 19.75) -> (22, 26.4055) projected
  arc A0 (22, 26.4055) -> (-22, 26.4055) centre (0, 0) ccw projected
  line L2 (-22, 26.4055) -> (-22, 19.75) projected
  line L3 (17, 25.75) -> (-17, 25.75) projected
  line L4 (17, 24.25) -> (17, 25.75) projected
  line L5 (-17, 24.25) -> (17, 24.25) projected
  line L6 (-17, 25.75) -> (-17, 24.25) projected
  line L7 (20.5, 22.75) -> (-20.5, 22.75) projected
  line L8 (20.5, 21.25) -> (20.5, 22.75) projected
  line L9 (-20.5, 21.25) -> (20.5, 21.25) projected
  line L10 (-20.5, 22.75) -> (-20.5, 21.25) projected
  line L11 (-22, 10.75) -> (-17, 10.75) projected
  line L12 (-2.5, 10.75) -> (-17, 10.75) projected
  line L13 (-2.5, 10.75) -> (2.5, 10.75) projected
  line L14 (17, 10.75) -> (2.5, 10.75) projected
  line L15 (17, 10.75) -> (22, 10.75) projected
  line L16 (22, 19.75) -> (22, 10.75) projected
  line L17 (22, 19.75) -> (-22, 19.75) projected
  line L18 (-22, 10.75) -> (-22, 19.75) projected
  line L19 (-17, 10.75) -> (-22, 10.75) projected
  line L20 (-22, 10.75) -> (-22, 7.75) projected
  line L21 (-17, 7.75) -> (-22, 7.75) projected
  line L22 (-17, 7.75) -> (-17, 10.75) projected
  line L23 (-17, 5.25) -> (-17, 7.75) projected
  line L24 (-17, 7.75) -> (-22, 7.75) projected
  line L25 (-22, 5.25) -> (-22, 7.75) projected
  line L26 (-17, 5.25) -> (-22, 5.25) projected
  line L27 (2.5, 10.75) -> (-2.5, 10.75) projected
  line L28 (-2.5, 10.75) -> (-2.5, 7.75) projected
  line L29 (2.5, 7.75) -> (-2.5, 7.75) projected
  line L30 (2.5, 7.75) -> (2.5, 10.75) projected
  line L31 (2.5, 5.25) -> (2.5, 7.75) projected
  line L32 (2.5, 7.75) -> (-2.5, 7.75) projected
  line L33 (-2.5, 7.75) -> (-2.5, 5.25) projected
  line L34 (2.5, 5.25) -> (-2.5, 5.25) projected
  line L35 (22, 10.75) -> (17, 10.75) projected
  line L36 (17, 10.75) -> (17, 7.75) projected
  line L37 (22, 7.75) -> (17, 7.75) projected
  line L38 (22, 7.75) -> (22, 10.75) projected
  line L39 (17, 7.75) -> (17, 5.25) projected
  line L40 (22, 5.25) -> (17, 5.25) projected
  line L41 (22, 5.25) -> (22, 7.75) projected
  line L42 (22, 7.75) -> (17, 7.75) projected
  line L43 (-21.5, 5.25) -> (21.5, 5.25)
  line L44 (21.5, 5.25) -> (21.5, 34.3693)
  line L45 (21.5, 34.3693) -> (-21.5, 34.3693)
  line L46 (-21.5, 34.3693) -> (-21.5, 5.25)
  circle A1 centre (0, 0) radius 34.3693
  line L47 (-17, 5.25) -> (-22, 5.25) projected
  line L48 (-22, 5.25) -> (22, 5.25)
  line L49 (22, 5.25) -> (22, 35.1173)
  line L50 (22, 35.1173) -> (-22, 35.1173)
  line L51 (-22, 35.1173) -> (-22, 5.25)
  line L52 (-2, 10.75) -> (2, 10.75)
  line L53 (2, 10.75) -> (2, 5.25)
  line L54 (2, 5.25) -> (-2, 5.25)
  line L55 (-2, 5.25) -> (-2, 10.75)
  line L56 (-17, 5.25) -> (-17.5, 5.25)
  line L57 (-17.5, 5.25) -> (-17.5, 10.75)
  line L58 (-17.5, 10.75) -> (-17, 10.75)
  line L59 (-17, 10.75) -> (-17, 5.25)
  line L60 (17, 5.25) -> (17.5, 5.25)
  line L61 (17.5, 5.25) -> (17.5, 10.75)
  line L62 (17.5, 10.75) -> (17, 10.75)
  line L63 (17, 10.75) -> (17, 5.25)
  point P0 (21.5, 5.25)
  point P1 (21.5, 26.8142)
  point P2 (2, 10.75)
  point P3 (-2.5, 7.75)
  point P4 (-21.5, 26.8142)
  point P5 (-21.5, 5.25)
  dimension "d396" = 0
  dimension "d397" = 0.5
  dimension "d398" = 0.5
  dimension "d399" = 0.5
  dimension "d400" = 0.5
  dimension "d401" = 0
  dimension "d402" = 0
  dimension "d410" = 0.5
  dimension "d411" = 0.5
  constraints: 40 end point, 11 parallel, 5 horizontal, 5 perpendicular, 2 tangent, 1 centre point, 1 coincident, 1 collinear, 1 point on line
  measures "d396" distance between parallel lines of L43 L40
  measures "d397" distance between parallel lines of L44 L16
  measures "d398" distance between parallel lines of L18 L46
  measures "d399" distance between parallel lines of L53 L30
  measures "d400" distance between parallel lines of L28 L55
  measures "d401" distance between parallel lines of L13 L52
  measures "d402" distance between parallel lines of L34 L54
  measures "d410" distance between parallel lines of L57 L23
  measures "d411" distance between parallel lines of L39 L61
extrude "サイドがばがば用押し出し" cut sketch "がばがば用スケッチ" against normal blind 30 contours L2 A0 L46 L0 | L0 L46 L11 L18 | L11 L46 L21 L20 | L44 A0 L1 L0 | L0 L16 L15 L44 | L21 L46 L26 L25 | L15 L38 L37 L44 | L37 L41 L40 L44 | L13 L55 L29 L28 | L30 L29 L53 L13 | L29 L55 L34 L33 | L31 L34 L53 L29
extrude "サイドがばがば用押し出し２" cut sketch "がばがば用スケッチ" against normal blind 30 contours L11 L22 L21 L57 | L61 L37 L36 L15 | L21 L23 L26 L57 | L61 L40 L39 L37
sketch "スケッチ80" plane through (0, 0, 10.75) normal (0, 0, -1) x (-1, 0, 0)
  circle A0 centre (-7.25, 30) radius 1.25
  line L0 (-2, 37.0768) -> (-2, 20) projected
  line L1 (-2, 20) -> (-17, 20) projected
  point P0 (0, 0)
  dimension "d405" = 2.5
  dimension "d406" = 4
  dimension "d407" = 10
  constraints: 1 centre point
  measures "d405" diameter of A0
  measures "d406" distance edge to line of A0 L0
  measures "d407" distance from line of A0.centre L1
extrude "止めるようの穴" cut sketch "スケッチ80" against normal blind 30
